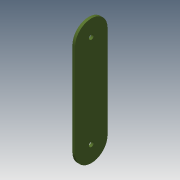
# Autodesk Inventor part: dibond2
Saved by Autodesk Inventor 2013 (Build 170138000, 138)
## iProperties
Created: 2013-01-30
Part Number: dibond2
Material: Generic
Document SubType Name: Modeling
Designer: idle-rug
Density: 1 g/cm^3
Author: idle-rug
Autodesk Inventor part; units mm, degrees
ref_plane "YZ Plane" through (0, 0, 0) normal (1, 0, 0) x (0, 1, 0)
ref_plane "XZ Plane" through (0, 0, 0) normal (0, 1, 0) x (-1, 0, 0)
ref_plane "XY Plane" through (0, 0, 0) normal (0, 0, 1) x (1, 0, 0)
sketch "Sketch1" plane through (0, 0, 0) normal (1, 0, 0) x (0, 1, 0)
  line L0 (21, -60) -> (-21, -60)
  line L1 (-21, -60) -> (-21, 60)
  line L2 (-21, 60) -> (21, 60)
  line L3 (21, 60) -> (21, -60)
  line L4 (21, -60) -> (-21, 60) construction
  line L5 (-21, -60) -> (21, 60) construction
  circle A0 centre (0, 60) radius 21
  circle A1 centre (0, -60) radius 21
  point P0 (0, 0)
  dimension "d0" = 42
  dimension "d1" = 120
  dimension "d2" = 42
  dimension "d3" = 42
  constraints: 12 end point, 4 midpoint, 2 centre point, 2 parallel, 1 horizontal, 1 perpendicular
  measures "d0" distance of L1.end L2.end
  measures "d1" distance of L0.end L1.end
  measures "d2" diameter of A0
  measures "d3" diameter of A1
extrude "Extrusion1" add sketch "Sketch1" along normal blind 3.4
sketch "Sketch2" plane through (3.4, 0, 0) normal (1, 0, 0) x (0, 0, -1)
  arc A0 (60, -21) -> (60, 21) centre (60, 0) ccw projected
  arc A1 (-60, 21) -> (-60, -21) centre (-60, 0) ccw projected
  circle A2 centre (-60, 0) radius 3
  circle A3 centre (60, 0) radius 3
  point P0 (0, 0)
  dimension "d6" = 6
  dimension "d7" = 6
  constraints: 2 centre point, 2 coincident
  measures "d6" diameter of A2
  measures "d7" diameter of A3
extrude "Extrusion2" cut sketch "Sketch2" against normal blind 3.4
body "Solid1"
